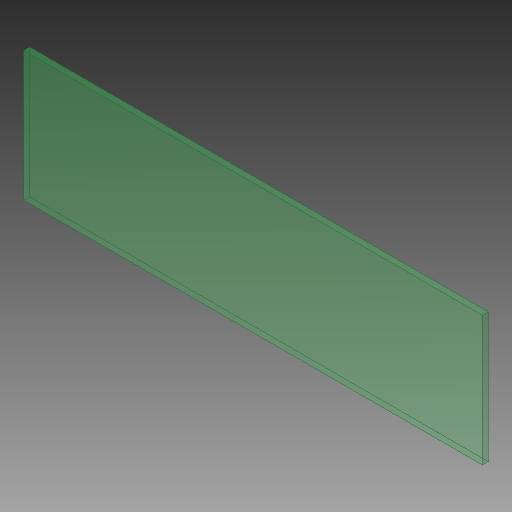
# Autodesk Inventor part: tank_bottom
Saved by Autodesk Inventor 2018.1 (Build 221171000, 171)
## iProperties
Created: 2017-07-30
Part Number: tank_bottom
Material: PVC-Piping
Document SubType Name: Modeling
Designer: Tom
Density: 1.4 g/cm^3
Appearance: Clear - Green 1
Mass: 236.477 g
Surface Area: 884.48 cm^2
Volume: 168.912 cm^3
Author: Tom
Autodesk Inventor part; units mm, degrees
ref_plane "YZ Plane" through (0, 0, 0) normal (1, 0, 0) x (0, 1, 0)
ref_plane "XZ Plane" through (0, 0, 0) normal (0, 1, 0) x (-1, 0, 0)
ref_plane "XY Plane" through (0, 0, 0) normal (0, 0, 1) x (1, 0, 0)
sketch "Sketch2" plane through (0, 0, 0) normal (0, 0, 1) x (1, 0, 0)
  line L0 (0, 0) -> (389, 0)
  line L1 (389, 0) -> (389, 110)
  line L2 (389, 110) -> (0, 110)
  line L3 (0, 110) -> (0, 0)
  dimension "d4" = 389
  dimension "d5" = 110
  constraints: 8 end point, 2 parallel, 1 horizontal, 1 perpendicular
  measures "d4" distance of L2.end L1.end
  measures "d5" distance of L1.end L0.end
extrude "Extrusion2" add sketch "Sketch2" along normal blind 5
equation "\"d4\" = tankl + 2 * pvct"
equation "\"d5\" = tankw + 2 * pvct"
equation "\"d6\" = pvct"
equation "\"lcsd\" = 19.05"
equation "\"lcwd1\" = 25"
equation "\"lcwd2\" = 34"
equation "\"lch1\" = 39"
equation "\"lcwd3\" = 43"
equation "\"dia1\" = 6"
equation "\"td\" = 18"
equation "\"bhh\" = 6"
equation "\"sw\" = 25"
equation "\"sh\" = 31"
equation "\"spacert\" = 2"
equation "\"pvct\" = 5"
equation "\"tankl\" = 379"
equation "\"dia3\" = 8"
equation "\"dia4\" = 11"
equation "\"play\" = 9"
equation "\"holeh\" = 26"
equation "\"slack\" = 0.5"
equation "\"surroundt\" = 5"
equation "\"play2\" = 3"
equation "\"diawater\" = 25"
equation "\"diaair\" = 32"
equation "\"diaoverflow\" = 25"
equation "\"diaph\" = 32"
equation "\"diacucl\" = 32"
equation "\"diasurroundhole\" = 42"
equation "\"diagrate\" = 12"
equation "\"gratespacing\" = 12.02082"
equation "\"bottomdist\" = 9.6355"
equation "\"sidedist\" = 13.9375"
equation "\"diahcl\" = 32"
equation "\"bracketwtop\" = 6"
equation "\"bracketwbottom\" = 6"
equation "\"nett\" = 1"
equation "\"nethole\" = 16"
equation "\"netside\" = 3.5"
equation "\"nettop\" = 7"
equation "\"netholespacing\" = 2"
equation "\"diaetape\" = 32"
equation "\"tankw\" = 100"
body "Solid2"
